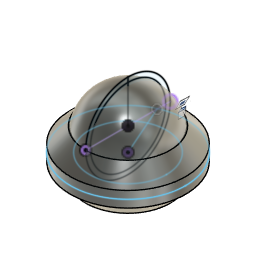
2025_04_14_ForFunWheelShip (Autodesk Fusion 360 design; units mm, degrees)
Autodesk Fusion 360 part; units mm, degrees
note: some values were not read from the file. Set by a fixed rule: which sketch regions a step uses.
sketch "Sketch1" plane through (0, 0, 0) normal (0, 0, 1) x (1, 0, 0)
  circle A0 centre (0, 0) radius 37.5718
  circle A1 centre (0, 0) radius 25.1296
  constraint coincident A0.centre A1.centre
  constraint concentric A0 A1
extrude "Extrude1" add sketch "Sketch1" along normal blind 10 contours A1 makes body 1
extrude "Extrude2" add sketch "Sketch1" along normal blind 15 bodies 1
mirror "Mirror1" about plane through (0, 0, 0) normal (0, 0, -1) of bodies 1 merged
chamfer "Chamfer1" distance 10 angle 45 2 edges at (-35.0292, -13.5865, 15) (-35.0292, -13.5865, -15) on bodies 1
sketch "Sketch2" plane through (0, 0, 0) normal (1, 0, 0) x (0, 1, 0)
  line L0 (-27.5718, 15) -> (27.5718, 15)
  line L1 (0, 0) -> (18.9639, 15)
  circle A0 centre (0, 15) radius 27.5718
  line L2 (0, 15) -> (0, 42.5718)
  circle A1 centre (0, 15) radius 24.5718
  point P0 (0, 15)
  dimension "d9" = -3
  constraint coincident L1.start origin
  constraint coincident L0 L1.end
  constraint coincident P0 A0.centre
  constraint coincident L0.start A0
  constraint coincident A0 L2.end
  constraint perpendicular L0 L2
revolve "Revolve1" add sketch "Sketch2" angle 360 about axis through (0, 0, 15) along (0, 0, 1) separate body contours L0 A0 L2 A1 picked at (-2.4736, 41.3948) makes body 2
move_body "Move1" bodies 2 to x (1, 0, 0) y (0, 1, 0) z (0, 0, 1) at (0, 0, -5)
